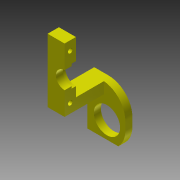
# Autodesk Inventor part: Part14
Saved by Autodesk Inventor 2015 (Build 190159000, 159)
## iProperties
Created: 2015-07-08
Part Number: Part14
Material: ABS Plastic
Document SubType Name: Modeling
Designer: eefred
Density: 1.06 g/cm^3
Appearance: Smooth - Yellow
Author: eefred
Autodesk Inventor part; units mm, degrees
ref_plane "YZ Plane" through (0, 0, 0) normal (1, 0, 0) x (0, 1, 0)
ref_plane "XZ Plane" through (0, 0, 0) normal (0, 1, 0) x (-1, 0, 0)
ref_plane "XY Plane" through (0, 0, 0) normal (0, 0, 1) x (1, 0, 0)
sketch "Sketch1" plane through (0, 0, 0) normal (0, 1, 0) x (-1, 0, 0)
  line L0 (0, 22.5) -> (12, 22.5)
  line L1 (12, 22.5) -> (12, -22.5)
  line L2 (12, -22.5) -> (0, -22.5)
  arc A0 (0, -6.15) -> (0, 6.15) centre (0, 0) ccw
  line L3 (0, 22.5) -> (0, 6.15)
  line L4 (0, -6.15) -> (0, -22.5)
  point P0 (12, 0)
  dimension "d0" = 12
  dimension "d1" = 45
  dimension "d2" = 6.15
  constraints: 10 end point, 3 coincident, 2 equal length, 2 point on circle, 2 vertical alignment, 1 centre point, 1 horizontal, 1 horizontal alignment, 1 midpoint, 1 perpendicular, 1 vertical
  measures "d0" distance of L1.end L2.end
  measures "d1" distance of L0.end L1.end
  measures "d2" radius of A0
extrude "Extrusion1" add sketch "Sketch1" along normal blind 8
sketch "Sketch2" plane through (0, 8, 0) normal (0, 1, 0) x (1, 0, 0)
  line L0 (0, -22.5) -> (0, -6.15) projected
  arc A0 (0, 7.65) -> (0, -7.65) centre (0, 0) ccw
  line L1 (0, -7.65) -> (0, 7.65)
  dimension "d5" = 7.65
  constraints: 2 end point, 2 point on circle, 1 centre point, 1 coincident, 1 point on line, 1 vertical
  measures "d5" radius of A0
extrude "Extrusion2" cut sketch "Sketch2" against normal blind 3
sketch "Sketch3" plane through (0, 0, 22.5) normal (1, 0, 0) x (0, 0, -1)
  circle A0 centre (6.5, 4) radius 1.6
  circle A1 centre (38.5, 4) radius 1.6
  line L0 (16.35, 0) -> (0, 0) projected
  point P0 (22.5, 0)
  dimension "d8" = 3.2
  dimension "d9" = 32
  dimension "d10" = 4
  dimension "d11" = 16
  constraints: 2 centre point, 1 equal radius, 1 horizontal alignment
  measures "d8" diameter of A0
  measures "d9" distance of A1.centre A0.centre
  measures "d10" distance from line of L0 A0.centre
  measures "d11" horizontal distance of point (22.5, 0) A0.centre
extrude "Extrusion3" cut sketch "Sketch3" against normal up to next
sketch "Sketch4" plane through (0, 8, 0) normal (0, 1, 0) x (1, 0, 0)
  line L0 (-12, 22.5) -> (0, 22.5)
  line L1 (0, 22.5) -> (0, 14.5)
  line L2 (0, 14.5) -> (-12, 14.5)
  line L3 (-12, 14.5) -> (-12, 22.5)
  point P0 (0, 0)
  dimension "d14" = 8
  constraints: 8 end point, 2 parallel, 1 horizontal, 1 perpendicular
  measures "d14" distance of L0.end L1.end
extrude "Extrusion4" add sketch "Sketch4" along normal blind 20
sketch "Sketch5" plane through (0, 28, 0) normal (0, 1, 0) x (1, 0, 0)
  line L0 (10.0416, 49.5) -> (-12, 49.5)
  line L1 (-12, 49.5) -> (-12, 14.5)
  arc A0 (-2, 14.5) -> (15, 31.5) centre (-2, 31.5) ccw
  line L2 (-12, 14.5) -> (-2, 14.5)
  line L3 (15, 31.5) -> (15, 37.5)
  arc A1 (15, 37.5) -> (10.0416, 49.5) centre (-2, 37.5) ccw
  circle A2 centre (2, 37.5) radius 9.3
  point P0 (0, 0)
  dimension "d19" = 35
  dimension "d20" = 17
  dimension "d21" = 10
  dimension "d22" = 6
  dimension "d23" = 18.6
  dimension "d24" = 14
  constraints: 8 end point, 4 point on circle, 3 centre point, 3 tangent, 2 horizontal, 2 vertical, 1 horizontal alignment, 1 vertical alignment
  measures "d19" distance of L0.end L1.end
  measures "d20" radius of A0
  measures "d21" distance from line of L1 A0.centre
  measures "d22" distance of A1.centre A0.centre
  measures "d23" diameter of A2
  measures "d24" distance from line of L1 A2.centre
extrude "Extrusion5" add sketch "Sketch5" along normal blind 5
equation "\"d11\" = 0.5 * d9"
body "Solid1"
